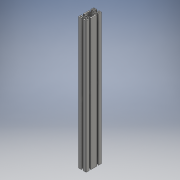
# Autodesk Inventor part: 240628_final5(680)
Saved by Autodesk Inventor 2016 (Build 200138000, 138)
## iProperties
Created: 2024-06-28
Part Number: 240628_final5(680)
Material: 일반
Document SubType Name: Modeling
Designer: pc
Density: 1 g/cm^3
Appearance: 기본값
Author: pc
Autodesk Inventor part; units mm, degrees
ref_plane "YZ Plane" through (0, 0, 0) normal (1, 0, 0) x (0, 1, 0)
ref_plane "XZ Plane" through (0, 0, 0) normal (0, 1, 0) x (-1, 0, 0)
ref_plane "XY Plane" through (0, 0, 0) normal (0, 0, 1) x (1, 0, 0)
sketch "스케치1" plane through (0, 0, 0) normal (0, 0, 1) x (1, 0, 0)
  line L0 (3.2869, -33.8744) -> (3.2869, -36.8744)
  arc A0 (3.2869, -36.8744) -> (3.7869, -37.3744) centre (3.7869, -36.8744) ccw
  line L1 (3.7869, -37.3744) -> (17.1433, -37.3744)
  line L2 (17.1433, -37.3744) -> (18.1433, -37.3744)
  arc A1 (18.1433, -37.3744) -> (19.1433, -36.3744) centre (18.1433, -36.3744) ccw
  line L3 (19.1433, -36.3744) -> (19.1433, -35.3744)
  line L4 (19.1433, -35.3744) -> (19.1433, -22.018)
  arc A2 (19.1433, -22.018) -> (18.6433, -21.518) centre (18.6433, -22.018) ccw
  line L5 (18.6433, -21.518) -> (15.6433, -21.518)
  arc A3 (15.6433, -21.518) -> (15.1433, -22.018) centre (15.6433, -22.018) ccw
  line L6 (15.1433, -22.018) -> (15.1433, -24.022)
  arc A4 (14.6433, -24.522) -> (15.1433, -24.022) centre (14.6433, -24.022) ccw
  line L7 (14.6433, -24.522) -> (8.5762, -24.522)
  arc A5 (8.2392, -24.3913) -> (8.5762, -24.522) centre (8.5762, -24.022) ccw
  arc A6 (5.1572, -17.8883) -> (8.2392, -24.3913) centre (14.6433, -17.3744) ccw
  line L8 (5.1572, -17.8883) -> (4.6433, -17.3744)
  line L9 (4.6433, -17.3744) -> (5.1572, -16.8605)
  arc A7 (8.2392, -10.3575) -> (5.1572, -16.8605) centre (14.6433, -17.3744) ccw
  arc A8 (8.5762, -10.2268) -> (8.2392, -10.3575) centre (8.5762, -10.7268) ccw
  line L10 (8.5762, -10.2268) -> (14.6433, -10.2268)
  arc A9 (15.1433, -10.7268) -> (14.6433, -10.2268) centre (14.6433, -10.7268) ccw
  line L11 (15.1433, -10.7268) -> (15.1433, -12.7309)
  arc A10 (15.1433, -12.7309) -> (15.6433, -13.2309) centre (15.6433, -12.7309) ccw
  line L12 (15.6433, -13.2309) -> (18.6433, -13.2309)
  arc A11 (18.6433, -13.2309) -> (19.1433, -12.7309) centre (18.6433, -12.7309) ccw
  line L13 (19.1433, -12.7309) -> (19.1433, 17.982)
  arc A12 (19.1433, 17.982) -> (18.6433, 18.482) centre (18.6433, 17.982) ccw
  line L14 (18.6433, 18.482) -> (15.6433, 18.482)
  arc A13 (15.6433, 18.482) -> (15.1433, 17.982) centre (15.6433, 17.982) ccw
  line L15 (15.1433, 17.982) -> (15.1433, 15.978)
  arc A14 (14.6433, 15.478) -> (15.1433, 15.978) centre (14.6433, 15.978) ccw
  line L16 (14.6433, 15.478) -> (8.5762, 15.478)
  arc A15 (8.2392, 15.6087) -> (8.5762, 15.478) centre (8.5762, 15.978) ccw
  arc A16 (5.1572, 22.1117) -> (8.2392, 15.6087) centre (14.6433, 22.6256) ccw
  line L17 (5.1572, 22.1117) -> (4.6433, 22.6256)
  line L18 (4.6433, 22.6256) -> (5.1572, 23.1395)
  arc A17 (8.2392, 29.6425) -> (5.1572, 23.1395) centre (14.6433, 22.6256) ccw
  arc A18 (8.5762, 29.7732) -> (8.2392, 29.6425) centre (8.5762, 29.2732) ccw
  line L19 (8.5762, 29.7732) -> (14.6433, 29.7732)
  arc A19 (15.1433, 29.2732) -> (14.6433, 29.7732) centre (14.6433, 29.2732) ccw
  line L20 (15.1433, 29.2732) -> (15.1433, 27.2691)
  arc A20 (15.1433, 27.2691) -> (15.6433, 26.7691) centre (15.6433, 27.2691) ccw
  line L21 (15.6433, 26.7691) -> (18.6433, 26.7691)
  arc A21 (18.6433, 26.7691) -> (19.1433, 27.2691) centre (18.6433, 27.2691) ccw
  line L22 (19.1433, 27.2691) -> (19.1433, 40.6256)
  line L23 (19.1433, 40.6256) -> (19.1433, 41.6256)
  arc A22 (19.1433, 41.6256) -> (18.1433, 42.6256) centre (18.1433, 41.6256) ccw
  line L24 (18.1433, 42.6256) -> (17.1433, 42.6256)
  line L25 (17.1433, 42.6256) -> (3.7869, 42.6256)
  arc A23 (3.7869, 42.6256) -> (3.2869, 42.1256) centre (3.7869, 42.1256) ccw
  line L26 (3.2869, 42.1256) -> (3.2869, 39.1256)
  arc A24 (3.2869, 39.1256) -> (3.7869, 38.6256) centre (3.7869, 39.1256) ccw
  line L27 (3.7869, 38.6256) -> (5.7909, 38.6256)
  arc A25 (6.2909, 38.1256) -> (5.7909, 38.6256) centre (5.7909, 38.1256) ccw
  line L28 (6.2909, 38.1256) -> (6.2909, 32.0585)
  arc A26 (6.1602, 31.7214) -> (6.2909, 32.0585) centre (5.7909, 32.0585) ccw
  arc A27 (-0.3428, 28.6395) -> (6.1602, 31.7214) centre (-0.8567, 38.1256) ccw
  line L29 (-0.3428, 28.6395) -> (-0.8567, 28.1256)
  line L30 (-0.8567, 28.1256) -> (-1.3706, 28.6395)
  arc A28 (-7.8736, 31.7214) -> (-1.3706, 28.6395) centre (-0.8567, 38.1256) ccw
  arc A29 (-8.0043, 32.0585) -> (-7.8736, 31.7214) centre (-7.5043, 32.0585) ccw
  line L31 (-8.0043, 32.0585) -> (-8.0043, 38.1256)
  arc A30 (-7.5043, 38.6256) -> (-8.0043, 38.1256) centre (-7.5043, 38.1256) ccw
  line L32 (-7.5043, 38.6256) -> (-5.5003, 38.6256)
  arc A31 (-5.5003, 38.6256) -> (-5.0003, 39.1256) centre (-5.5003, 39.1256) ccw
  line L33 (-5.0003, 39.1256) -> (-5.0003, 42.1256)
  arc A32 (-5.0003, 42.1256) -> (-5.5003, 42.6256) centre (-5.5003, 42.1256) ccw
  line L34 (-5.5003, 42.6256) -> (-18.8567, 42.6256)
  line L35 (-18.8567, 42.6256) -> (-19.8567, 42.6256)
  arc A33 (-19.8567, 42.6256) -> (-20.8567, 41.6256) centre (-19.8567, 41.6256) ccw
  line L36 (-20.8567, 41.6256) -> (-20.8567, 40.6256)
  line L37 (-20.8567, 40.6256) -> (-20.8567, 27.2691)
  arc A34 (-20.8567, 27.2691) -> (-20.3567, 26.7691) centre (-20.3567, 27.2691) ccw
  line L38 (-20.3567, 26.7691) -> (-17.3567, 26.7691)
  arc A35 (-17.3567, 26.7691) -> (-16.8567, 27.2691) centre (-17.3567, 27.2691) ccw
  line L39 (-16.8567, 27.2691) -> (-16.8567, 29.2732)
  arc A36 (-16.3567, 29.7732) -> (-16.8567, 29.2732) centre (-16.3567, 29.2732) ccw
  line L40 (-16.3567, 29.7732) -> (-10.2896, 29.7732)
  arc A37 (-9.9526, 29.6425) -> (-10.2896, 29.7732) centre (-10.2896, 29.2732) ccw
  arc A38 (-6.8706, 23.1395) -> (-9.9526, 29.6425) centre (-16.3567, 22.6256) ccw
  line L41 (-6.8706, 23.1395) -> (-6.3567, 22.6256)
  line L42 (-6.3567, 22.6256) -> (-6.8706, 22.1117)
  arc A39 (-9.9526, 15.6087) -> (-6.8706, 22.1117) centre (-16.3567, 22.6256) ccw
  arc A40 (-10.2896, 15.478) -> (-9.9526, 15.6087) centre (-10.2896, 15.978) ccw
  line L43 (-10.2896, 15.478) -> (-16.3567, 15.478)
  arc A41 (-16.8567, 15.978) -> (-16.3567, 15.478) centre (-16.3567, 15.978) ccw
  line L44 (-16.8567, 15.978) -> (-16.8567, 17.982)
  arc A42 (-16.8567, 17.982) -> (-17.3567, 18.482) centre (-17.3567, 17.982) ccw
  line L45 (-17.3567, 18.482) -> (-20.3567, 18.482)
  arc A43 (-20.3567, 18.482) -> (-20.8567, 17.982) centre (-20.3567, 17.982) ccw
  line L46 (-20.8567, 17.982) -> (-20.8567, -12.7309)
  arc A44 (-20.8567, -12.7309) -> (-20.3567, -13.2309) centre (-20.3567, -12.7309) ccw
  line L47 (-20.3567, -13.2309) -> (-17.3567, -13.2309)
  arc A45 (-17.3567, -13.2309) -> (-16.8567, -12.7309) centre (-17.3567, -12.7309) ccw
  line L48 (-16.8567, -12.7309) -> (-16.8567, -10.7268)
  arc A46 (-16.3567, -10.2268) -> (-16.8567, -10.7268) centre (-16.3567, -10.7268) ccw
  line L49 (-16.3567, -10.2268) -> (-10.2896, -10.2268)
  arc A47 (-9.9526, -10.3575) -> (-10.2896, -10.2268) centre (-10.2896, -10.7268) ccw
  arc A48 (-6.8706, -16.8605) -> (-9.9526, -10.3575) centre (-16.3567, -17.3744) ccw
  line L50 (-6.8706, -16.8605) -> (-6.3567, -17.3744)
  line L51 (-6.3567, -17.3744) -> (-6.8706, -17.8883)
  arc A49 (-9.9526, -24.3913) -> (-6.8706, -17.8883) centre (-16.3567, -17.3744) ccw
  arc A50 (-10.2896, -24.522) -> (-9.9526, -24.3913) centre (-10.2896, -24.022) ccw
  line L52 (-10.2896, -24.522) -> (-16.3567, -24.522)
  arc A51 (-16.8567, -24.022) -> (-16.3567, -24.522) centre (-16.3567, -24.022) ccw
  line L53 (-16.8567, -24.022) -> (-16.8567, -22.018)
  arc A52 (-16.8567, -22.018) -> (-17.3567, -21.518) centre (-17.3567, -22.018) ccw
  line L54 (-17.3567, -21.518) -> (-20.3567, -21.518)
  arc A53 (-20.3567, -21.518) -> (-20.8567, -22.018) centre (-20.3567, -22.018) ccw
  line L55 (-20.8567, -22.018) -> (-20.8567, -35.3744)
  line L56 (-20.8567, -35.3744) -> (-20.8567, -36.3744)
  arc A54 (-20.8567, -36.3744) -> (-19.8567, -37.3744) centre (-19.8567, -36.3744) ccw
  line L57 (-19.8567, -37.3744) -> (-18.8567, -37.3744)
  line L58 (-18.8567, -37.3744) -> (-5.5003, -37.3744)
  arc A55 (-5.5003, -37.3744) -> (-5.0003, -36.8744) centre (-5.5003, -36.8744) ccw
  line L59 (-5.0003, -36.8744) -> (-5.0003, -33.8744)
  arc A56 (-5.0003, -33.8744) -> (-5.5003, -33.3744) centre (-5.5003, -33.8744) ccw
  line L60 (-5.5003, -33.3744) -> (-7.5043, -33.3744)
  arc A57 (-8.0043, -32.8744) -> (-7.5043, -33.3744) centre (-7.5043, -32.8744) ccw
  line L61 (-8.0043, -32.8744) -> (-8.0043, -26.8074)
  arc A58 (-7.8736, -26.4703) -> (-8.0043, -26.8074) centre (-7.5043, -26.8074) ccw
  arc A59 (-1.3706, -23.3883) -> (-7.8736, -26.4703) centre (-0.8567, -32.8744) ccw
  line L62 (-1.3706, -23.3883) -> (-0.8567, -22.8744)
  line L63 (-0.8567, -22.8744) -> (-0.3428, -23.3883)
  arc A60 (6.1602, -26.4703) -> (-0.3428, -23.3883) centre (-0.8567, -32.8744) ccw
  arc A61 (6.2909, -26.8074) -> (6.1602, -26.4703) centre (5.7909, -26.8074) ccw
  line L64 (6.2909, -26.8074) -> (6.2909, -32.8744)
  arc A62 (5.7909, -33.3744) -> (6.2909, -32.8744) centre (5.7909, -32.8744) ccw
  line L65 (5.7909, -33.3744) -> (3.7869, -33.3744)
  arc A63 (3.7869, -33.3744) -> (3.2869, -33.8744) centre (3.7869, -33.8744) ccw
  circle A64 centre (12.6433, 36.1256) radius 4
  line L66 (1.3495, 19.7196) -> (2.0424, 19.021)
  arc A65 (2.0424, 19.021) -> (2.4676, 19.0202) centre (2.2554, 19.2323) ccw
  line L67 (2.4676, 19.0202) -> (2.7487, 19.3013)
  arc A66 (2.7487, 19.3013) -> (2.7478, 19.7264) centre (2.5365, 19.5134) ccw
  line L68 (2.7478, 19.7264) -> (2.0492, 20.4194)
  arc A67 (2.0078, 20.794) -> (2.0492, 20.4194) centre (2.2605, 20.6324) ccw
  arc A68 (2.0078, 20.794) -> (2.0078, 24.4572) centre (-0.8567, 22.6256) ccw
  arc A69 (2.0492, 24.8318) -> (2.0078, 24.4572) centre (2.2605, 24.6188) ccw
  line L69 (2.0492, 24.8318) -> (2.7478, 25.5247)
  arc A70 (2.7478, 25.5247) -> (2.7487, 25.9498) centre (2.5365, 25.7377) ccw
  line L70 (2.7487, 25.9498) -> (2.4676, 26.2309)
  arc A71 (2.4676, 26.2309) -> (2.0424, 26.2301) centre (2.2554, 26.0188) ccw
  line L71 (2.0424, 26.2301) -> (1.3495, 25.5315)
  arc A72 (0.9749, 25.49) -> (1.3495, 25.5315) centre (1.1365, 25.7428) ccw
  arc A73 (0.9749, 25.49) -> (-2.6883, 25.49) centre (-0.8567, 22.6256) ccw
  arc A74 (-3.0629, 25.5315) -> (-2.6883, 25.49) centre (-2.8499, 25.7428) ccw
  line L72 (-3.0629, 25.5315) -> (-3.7559, 26.2301)
  arc A75 (-3.7559, 26.2301) -> (-4.181, 26.2309) centre (-3.9688, 26.0188) ccw
  line L73 (-4.181, 26.2309) -> (-4.4621, 25.9498)
  arc A76 (-4.4621, 25.9498) -> (-4.4612, 25.5247) centre (-4.25, 25.7377) ccw
  line L74 (-4.4612, 25.5247) -> (-3.7627, 24.8318)
  arc A77 (-3.7212, 24.4572) -> (-3.7627, 24.8318) centre (-3.9739, 24.6188) ccw
  arc A78 (-3.7212, 24.4572) -> (-3.7212, 20.794) centre (-0.8567, 22.6256) ccw
  arc A79 (-3.7627, 20.4194) -> (-3.7212, 20.794) centre (-3.9739, 20.6324) ccw
  line L75 (-3.7627, 20.4194) -> (-4.4612, 19.7264)
  arc A80 (-4.4612, 19.7264) -> (-4.4621, 19.3013) centre (-4.25, 19.5134) ccw
  line L76 (-4.4621, 19.3013) -> (-4.181, 19.0202)
  arc A81 (-4.181, 19.0202) -> (-3.7559, 19.021) centre (-3.9688, 19.2323) ccw
  line L77 (-3.7559, 19.021) -> (-3.0629, 19.7196)
  arc A82 (-2.6883, 19.7611) -> (-3.0629, 19.7196) centre (-2.8499, 19.5083) ccw
  arc A83 (-2.6883, 19.7611) -> (0.9749, 19.7611) centre (-0.8567, 22.6256) ccw
  arc A84 (1.3495, 19.7196) -> (0.9749, 19.7611) centre (1.1365, 19.5083) ccw
  circle A85 centre (-14.3567, 36.1256) radius 4
  arc A86 (-4.9446, -11.2866) -> (-4.7324, -11.3744) centre (-4.7324, -11.0744) ccw
  line L78 (-4.9446, -11.2866) -> (-8.8567, -7.3744)
  line L79 (-8.8567, -7.3744) -> (-12.8567, -7.3744)
  arc A87 (-15.8567, -4.3744) -> (-12.8567, -7.3744) centre (-12.8567, -4.3744) ccw
  line L80 (-15.8567, -4.3744) -> (-15.8567, 9.6256)
  arc A88 (-12.8567, 12.6256) -> (-15.8567, 9.6256) centre (-12.8567, 9.6256) ccw
  line L81 (-12.8567, 12.6256) -> (-8.8567, 12.6256)
  line L82 (-8.8567, 12.6256) -> (-4.9446, 16.5377)
  arc A89 (-4.7324, 16.6256) -> (-4.9446, 16.5377) centre (-4.7324, 16.3256) ccw
  line L83 (-4.7324, 16.6256) -> (3.019, 16.6256)
  arc A90 (3.2312, 16.5377) -> (3.019, 16.6256) centre (3.019, 16.3256) ccw
  line L84 (3.2312, 16.5377) -> (7.1433, 12.6256)
  line L85 (7.1433, 12.6256) -> (11.1433, 12.6256)
  arc A91 (14.1433, 9.6256) -> (11.1433, 12.6256) centre (11.1433, 9.6256) ccw
  line L86 (14.1433, 9.6256) -> (14.1433, -4.3744)
  arc A92 (11.1433, -7.3744) -> (14.1433, -4.3744) centre (11.1433, -4.3744) ccw
  line L87 (11.1433, -7.3744) -> (7.1433, -7.3744)
  line L88 (7.1433, -7.3744) -> (3.2312, -11.2866)
  arc A93 (3.019, -11.3744) -> (3.2312, -11.2866) centre (3.019, -11.0744) ccw
  line L89 (3.019, -11.3744) -> (-4.7324, -11.3744)
  line L90 (1.3495, -20.2804) -> (2.0424, -20.979)
  arc A94 (2.0424, -20.979) -> (2.4676, -20.9798) centre (2.2554, -20.7677) ccw
  line L91 (2.4676, -20.9798) -> (2.7487, -20.6987)
  arc A95 (2.7487, -20.6987) -> (2.7478, -20.2736) centre (2.5365, -20.4866) ccw
  line L92 (2.7478, -20.2736) -> (2.0492, -19.5806)
  arc A96 (2.0078, -19.206) -> (2.0492, -19.5806) centre (2.2605, -19.3676) ccw
  arc A97 (2.0078, -19.206) -> (2.0078, -15.5428) centre (-0.8567, -17.3744) ccw
  arc A98 (2.0492, -15.1682) -> (2.0078, -15.5428) centre (2.2605, -15.3812) ccw
  line L93 (2.0492, -15.1682) -> (2.7478, -14.4753)
  arc A99 (2.7478, -14.4753) -> (2.7487, -14.0502) centre (2.5365, -14.2623) ccw
  line L94 (2.7487, -14.0502) -> (2.4676, -13.7691)
  arc A100 (2.4676, -13.7691) -> (2.0424, -13.7699) centre (2.2554, -13.9812) ccw
  line L95 (2.0424, -13.7699) -> (1.3495, -14.4685)
  arc A101 (0.9749, -14.51) -> (1.3495, -14.4685) centre (1.1365, -14.2572) ccw
  arc A102 (0.9749, -14.51) -> (-2.6883, -14.51) centre (-0.8567, -17.3744) ccw
  arc A103 (-3.0629, -14.4685) -> (-2.6883, -14.51) centre (-2.8499, -14.2572) ccw
  line L96 (-3.0629, -14.4685) -> (-3.7559, -13.7699)
  arc A104 (-3.7559, -13.7699) -> (-4.181, -13.7691) centre (-3.9688, -13.9812) ccw
  line L97 (-4.181, -13.7691) -> (-4.4621, -14.0502)
  arc A105 (-4.4621, -14.0502) -> (-4.4612, -14.4753) centre (-4.25, -14.2623) ccw
  line L98 (-4.4612, -14.4753) -> (-3.7627, -15.1682)
  arc A106 (-3.7212, -15.5428) -> (-3.7627, -15.1682) centre (-3.9739, -15.3812) ccw
  arc A107 (-3.7212, -15.5428) -> (-3.7212, -19.206) centre (-0.8567, -17.3744) ccw
  arc A108 (-3.7627, -19.5806) -> (-3.7212, -19.206) centre (-3.9739, -19.3676) ccw
  line L99 (-3.7627, -19.5806) -> (-4.4612, -20.2736)
  arc A109 (-4.4612, -20.2736) -> (-4.4621, -20.6987) centre (-4.25, -20.4866) ccw
  line L100 (-4.4621, -20.6987) -> (-4.181, -20.9798)
  arc A110 (-4.181, -20.9798) -> (-3.7559, -20.979) centre (-3.9688, -20.7677) ccw
  line L101 (-3.7559, -20.979) -> (-3.0629, -20.2804)
  arc A111 (-2.6883, -20.2389) -> (-3.0629, -20.2804) centre (-2.8499, -20.4917) ccw
  arc A112 (-2.6883, -20.2389) -> (0.9749, -20.2389) centre (-0.8567, -17.3744) ccw
  arc A113 (1.3495, -20.2804) -> (0.9749, -20.2389) centre (1.1365, -20.4917) ccw
  circle A114 centre (-14.3567, -30.8744) radius 4
  circle A115 centre (12.6433, -30.8744) radius 4
  point P0 (0, 0)
  constraints: 224 point on circle, 204 end point, 116 centre point
extrude "돌출1" add sketch "스케치1" along normal blind 680
